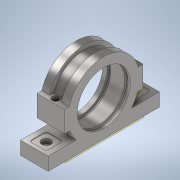
# Autodesk Inventor part: Корпус_Подшипника
Saved by Autodesk Inventor 2021 (Build 250183000, 183)
## iProperties
Created: 2023-04-25
Part Number: Корпус_Подшипника
Material: Сталь, углеродистая
Document SubType Name: Modeling
Designer: gdevc
Density: 7.85 g/cm^3
Appearance: С умеренной полировкой
Author: gdevc
Autodesk Inventor part; units mm, degrees
ref_plane "YZ Plane" through (0, 0, 0) normal (1, 0, 0) x (0, 1, 0)
ref_plane "XY Plane" through (0, 0, 0) normal (0, 0, 1) x (1, 0, 0)
sketch "Эскиз1" plane through (0, 0, 0) normal (0, 0, 1) x (1, 0, 0)
  line L0 (0, 0) -> (119.1589, 0)
  line L1 (0, 50) -> (52, 50)
  line L2 (52, 50) -> (52, 67.5)
  line L3 (0, 67.5) -> (0, 50)
  line L4 (0, 67.5) -> (15, 67.5)
  line L5 (15, 67.5) -> (15, 60)
  line L6 (15, 60) -> (37, 60)
  line L7 (37, 60) -> (37, 67.5)
  line L8 (37, 67.5) -> (52, 67.5)
  dimension "d0" = 100
  dimension "d1" = 52
  dimension "d2" = 135
  dimension "d3" = 10
  dimension "d4" = 15
  dimension "d5" = 15
  constraints: 18 end point, 5 perpendicular, 3 horizontal, 2 point on line
  measures "d0" diameter of L1 L0
  measures "d1" distance of L1.start L1.end
  measures "d2" diameter of L4 L0
  measures "d3" distance between parallel lines of L1 L6
  measures "d4" distance between parallel lines of L3 L5
  measures "d5" distance between parallel lines of L2 L7
revolve "Вращение1" add sketch "Эскиз1" angle 360 about axis through (0, 0, 0) along (1, 0, 0)
ref_plane "РабПлоскость1" through (0, -67.5, 0) normal (0, 1, 0) x (-1, 0, 0)
sketch "Эскиз3" plane through (0, -67.5, 0) normal (0, 1, 0) x (-1, 0, 0)
  line L0 (0, 0) -> (0, -105)
  line L1 (0, 67.5) -> (0, -67.5) projected
  line L2 (0, -105) -> (-52, -105)
  line L3 (-52, 67.5) -> (-52, -67.5) projected
  line L4 (-52, -105) -> (-52, 47.2217)
  line L5 (0, 105) -> (0, 0)
  line L6 (0, 105) -> (-52, 105)
  line L7 (-52, 105) -> (-52, 44.8764)
  dimension "d15" = 52
  dimension "d16" = 210
  dimension "d17" = 105
  constraints: 12 end point, 1 collinear, 1 horizontal, 1 parallel, 1 perpendicular, 1 point on line
  measures "d15" distance of L0.end L2.end
  measures "d16" distance between parallel lines of L6 L2
  measures "d17" distance from line of L0.start L2
extrude "Выдавливание1" add sketch "Эскиз3" along normal blind 25
sketch "Эскиз2" plane through (0, 0, 0) normal (0, 0, 1) x (1, 0, 0)
  line L0 (9, 50) -> (9, 54)
  line L1 (9, 54) -> (15, 54)
  line L2 (15, 54) -> (15, 50)
  line L3 (42, 50) -> (42, 54)
  line L4 (42, 54) -> (48, 54)
  line L5 (48, 54) -> (48, 50)
  line L6 (52, -67.5) -> (52, 67.5) projected
  line L7 (-10.4, 0) -> (62.4, 0) projected
  line L8 (15, 54) -> (15, 0)
  line L9 (15, -42.5) -> (15, 60) projected
  line L10 (9, 0) -> (9, 50)
  line L11 (48, 50) -> (48, 0)
  line L12 (48, 0) -> (42, 0)
  line L13 (42, 50) -> (42, 0)
  line L14 (52, 50) -> (0, 50) projected
  line L15 (9, 0) -> (15, 0)
  point P0 (0, 0)
  dimension "d7" = 54
  dimension "d8" = 6
  dimension "d9" = 9
  dimension "d10" = 4
  dimension "d11" = 54
  dimension "d12" = 6
  constraints: 24 end point, 5 perpendicular, 5 point on line, 2 vertical, 1 collinear
  measures "d7" distance from line of point (0, 0) L1
  measures "d8" distance between parallel lines of L2 L0
  measures "d9" distance from line of point (0, 0) L0
  measures "d10" distance between parallel lines of L6 L5
  measures "d11" distance from line of point (0, 0) L4
  measures "d12" distance between parallel lines of L5 L3
revolve "Вращение2" cut sketch "Эскиз2" angle 360 about axis through (-10, 0, 0) along (1, 0, 0) contours L14 L8 L7 L10 | L0 L1 L2 L14 | L14 L11 L7 L13 | L3 L4 L5 L14
sketch "Эскиз4" plane through (0, -67.5, -105) normal (-1, 0, 0) x (0, 0, 1)
  arc A0 (131.3391, 25) -> (78.6609, 25) centre (105, 67.5) ccw projected
  arc A1 (157.4404, 25) -> (52.5596, 25) centre (105, 67.5) ccw projected
  circle A2 centre (105, 67.5) radius 50
  point P0 (78.6609, 25)
  constraints: 1 centre point, 1 coincident
extrude "Выдавливание2" cut sketch "Эскиз4" against normal through all
ref_plane "РабПлоскость2" through (0, -42.5, 0) normal (0, 1, 0) x (-1, 0, 0)
sketch "Эскиз5" plane through (0, -42.5, 0) normal (0, 1, 0) x (-1, 0, 0)
  line L0 (-37, -98.5) -> (-15, -98.5)
  line L1 (-10, -93.5) -> (-10, -71.5)
  line L2 (-15, -66.5) -> (-37, -66.5)
  line L3 (-42, -71.5) -> (-42, -93.5)
  line L4 (-42, -82.5) -> (-10, -82.5) construction
  arc A0 (-42, -93.5) -> (-37, -98.5) centre (-37, -93.5) ccw
  arc A1 (-15, -98.5) -> (-10, -93.5) centre (-15, -93.5) ccw
  arc A2 (-10, -71.5) -> (-15, -66.5) centre (-15, -71.5) ccw
  arc A3 (-37, -66.5) -> (-42, -71.5) centre (-37, -71.5) ccw
  circle A4 centre (-26, -82.5) radius 8.5
  line L5 (-80.9956, 0) -> (7.5507, 0) construction
  line L6 (-37, 98.5) -> (-15, 98.5)
  line L7 (-10, 93.5) -> (-10, 71.5)
  line L8 (-15, 66.5) -> (-37, 66.5)
  line L9 (-42, 71.5) -> (-42, 93.5)
  line L10 (-42, 82.5) -> (-10, 82.5) construction
  arc A5 (-37, 98.5) -> (-42, 93.5) centre (-37, 93.5) ccw
  arc A6 (-10, 93.5) -> (-15, 98.5) centre (-15, 93.5) ccw
  arc A7 (-15, 66.5) -> (-10, 71.5) centre (-15, 71.5) ccw
  arc A8 (-42, 71.5) -> (-37, 66.5) centre (-37, 71.5) ccw
  circle A9 centre (-26, 82.5) radius 8.5
  point P0 (0, 0)
  dimension "d23" = 165
  dimension "d24" = 32
  dimension "d25" = 32
  dimension "d26" = 10
  dimension "d27" = 5
  dimension "d28" = 17
  constraints: 22 end point, 16 point on circle, 15 symmetric about line, 10 centre point, 8 tangent, 3 equal radius, 3 midpoint, 2 horizontal, 2 parallel, 1 perpendicular, 5 other
  measures "d23" diameter of point (0, 0) L4
  measures "d24" distance between parallel lines of L2 L0
  measures "d25" distance between parallel lines of L3 L1
  measures "d26" distance from line of point (0, 0) L1
  measures "d27" radius of A0
  measures "d28" diameter of A4
extrude "Выдавливание3" cut sketch "Эскиз5" against normal blind 1
extrude "Выдавливание4" cut sketch "Эскиз5" against normal through all contours A4 | A9
ref_plane "РабПлоскость3" through (26, -67.5, -105) normal (-1, 0, 0) x (0, 0, 1)
sketch "Эскиз6" plane through (26, -67.5, -105) normal (-1, 0, 0) x (0, 0, 1)
  line L0 (210, 0) -> (0, 0) projected
  line L1 (7.5, 15) -> (37.5, 15)
  line L2 (37.5, 15) -> (37.5, 0)
  line L3 (37.5, 0) -> (7.5, 0)
  line L4 (7.5, 0) -> (7.5, 15)
  line L5 (31, 24) -> (14, 24) projected
  line L6 (31, 0) -> (14, 0) projected
  line L7 (31, 0) -> (14, 0) projected
  line L8 (22.5, 0) -> (22.5, 18.5711) construction
  line L9 (105, 67.5) -> (105, 0) construction
  line L10 (0, 0) -> (210, 0)
  line L11 (202.5, 15) -> (172.5, 15)
  line L12 (172.5, 15) -> (172.5, 0)
  line L13 (202.5, 0) -> (202.5, 15)
  point P0 (202.5, 0)
  point P1 (7.5, 0)
  dimension "d34" = 30
  dimension "d35" = 30
  dimension "d36" = 15
  constraints: 20 end point, 6 symmetric about line, 2 midpoint, 2 parallel, 2 point on line, 1 horizontal, 1 perpendicular, 1 vertical
  measures "d34" distance between parallel lines of L2 L4
  measures "d35" diameter of L4 L8
  measures "d36" distance between parallel lines of L0 L1
extrude "Выдавливание5" cut sketch "Эскиз6" along normal mid plane 42
ref_plane "РабПлоскость4" through (0, 18.5, 0) normal (0, 1, 0) x (-1, 0, 0)
sketch "Эскиз9" plane through (0, -67.5, -105) normal (-1, 0, 0) x (0, 0, 1)
  line L0 (-42, 86) -> (252, 86) projected
  arc A0 (157.4404, 25) -> (52.5596, 25) centre (105, 67.5) ccw projected
  arc A1 (147.3527, 25) -> (62.6473, 25) centre (105, 67.5) ccw projected
  line L1 (40.0847, 86) -> (31, 86)
  line L2 (31, 86) -> (31, 46)
  line L3 (31, 46) -> (41.0156, 46)
  line L4 (7.5, 15) -> (37.5, 15) projected
  line L5 (31, 24) -> (14, 24) projected
  dimension "d46" = 40
  constraints: 6 end point, 3 point on line, 2 point on circle, 1 perpendicular, 1 vertical
  measures "d46" distance of L1.end L2.end
extrude "Выдавливание7" add sketch "Эскиз9" against normal blind 15 contours L0 A0 L3 L2
sketch "Эскиз10" plane through (26, -67.5, -105) normal (-1, 0, 0) x (0, 0, 1)
  line L0 (31, 46) -> (31, 86) projected
  line L1 (157.4404, 25) -> (147.3527, 25) projected
  arc A0 (147.3527, 25) -> (62.6473, 25) centre (105, 67.5) ccw projected
  line L2 (62.6473, 25) -> (52.5596, 25) projected
  arc A1 (41.0156, 46) -> (52.5596, 25) centre (105, 67.5) ccw projected
  line L3 (41.0156, 46) -> (31, 46) projected
  line L4 (31, 46) -> (31, 86) projected
  line L5 (31, 86) -> (40.0847, 86) projected
  arc A2 (157.4404, 25) -> (40.0847, 86) centre (105, 67.5) ccw projected
  arc A3 (147.3527, 25) -> (62.6473, 25) centre (105, 67.5) ccw projected
  line L6 (31, 86) -> (47.9233, 86)
  line L7 (31, 46) -> (41.0156, 46) projected
  line L8 (31, 46) -> (48.9844, 46)
  line L9 (105, 67.5) -> (105, 135) construction
  arc A4 (157.4404, 25) -> (40.0847, 86) centre (105, 67.5) ccw projected
  line L10 (179, 46) -> (179, 86)
  line L11 (168.9844, 46) -> (179, 46)
  line L12 (179, 46) -> (179, 86)
  line L13 (179, 86) -> (169.9153, 86)
  line L14 (179, 86) -> (162.0767, 86)
  line L15 (179, 46) -> (168.9844, 46)
  line L16 (179, 46) -> (161.0156, 46)
  point P0 (41.0156, 46)
  constraints: 20 end point, 8 symmetric about line, 3 point on circle, 1 collinear, 1 horizontal, 1 vertical
extrude "Выдавливание8" add sketch "Эскиз10" along normal mid plane 52 contours L0 L5 L6 A0 L8 L3 | L13 L10 L11 A2
ref_plane "РабПлоскость5" through (26, -67.5, 105) normal (1, 0, 0) x (0, 0, -1)
sketch "Эскиз11" plane through (26, -67.5, 105) normal (1, 0, 0) x (0, 0, -1)
  arc A0 (162.0767, 86) -> (62.6473, 25) centre (105, 67.5) ccw projected
  line L0 (31, 86) -> (40.0847, 86) projected
  line L1 (47.9233, 86) -> (31, 86)
  line L2 (31, 46) -> (31, 86) projected
  line L3 (31, 86) -> (31, 46)
  line L4 (31, 46) -> (48.9844, 46)
  arc A1 (47.9233, 86) -> (48.9844, 46) centre (105, 67.5) ccw
  constraints: 6 end point, 4 point on circle, 2 collinear, 1 centre point, 1 coincident, 1 perpendicular
extrude "Выдавливание9" add sketch "Эскиз11" along normal mid plane 52
sketch "Эскиз12" plane through (15, 18.5, -57.0767) normal (0, 1, 0) x (1, 0, 0)
  line L0 (0, 4.7941) -> (0, -1.0611) projected
  line L1 (22, -1.0611) -> (22, 6.9077) projected
  line L2 (-15, 16.9233) -> (37, 16.9233) projected
  line L3 (37, 6.9077) -> (37, 16.9233) projected
  line L4 (22, 6.9077) -> (37, 6.9077) projected
  line L5 (22, -1.0611) -> (22, 6.9077) projected
  line L6 (0, -1.0611) -> (22, -1.0611) projected
  line L7 (0, 6.9077) -> (0, -1.0611) projected
  line L8 (-15, 6.9077) -> (0, 6.9077) projected
  line L9 (0, -121.0611) -> (-15, -121.0611) projected
  line L10 (0, -113.0923) -> (0, -121.0611) projected
  line L11 (22, -113.0923) -> (0, -113.0923) projected
  line L12 (22, -121.0611) -> (22, -113.0923) projected
  line L13 (37, -121.0611) -> (22, -121.0611) projected
  circle A0 centre (11, 7.9389) radius 6.5
  line L14 (37, -107.0767) -> (37, -7.0767) projected
  line L15 (37, -57.0767) -> (-15, -57.0767) construction
  circle A1 centre (11, -122.0923) radius 6.5
  line L16 (37, -131.0767) -> (-15, -131.0767) projected
  line L17 (-15, -121.0611) -> (-15, -131.0767) projected
  line L18 (37, -131.0767) -> (37, -121.0611) projected
  line L19 (-15, 16.9233) -> (-15, 6.9077) projected
  dimension "d61" = 13
  dimension "d62" = 11
  dimension "d63" = 9
  constraints: 2 centre point, 2 end point, 1 horizontal, 1 midpoint, 1 symmetric about line, 1 other
  measures "d61" diameter of A0
  measures "d62" distance from line of L1 A0.centre
  measures "d63" distance from line of L6 A0.centre
ref_plane "РабПлоскость6" through (0, -21.5, -64.9153) normal (0, 1, 0) x (1, 0, 0)
sketch "Эскиз13" plane through (0, -21.5, -64.9153) normal (0, 1, 0) x (1, 0, 0)
  circle A0 centre (26, 0.1003) radius 6.5 projected
  circle A1 centre (26, -129.931) radius 6.5 projected
  circle A2 centre (26, 0.1003) radius 6
  circle A3 centre (26, -129.931) radius 6
  point P0 (0, -64.9153)
  dimension "d65" = 12
  dimension "d66" = 12
  constraints: 2 centre point, 2 coincident
  measures "d65" diameter of A2
  measures "d66" diameter of A3
extrude "Выдавливание10" cut sketch "Эскиз13" along normal blind 10 contours A2 | A3
thread "Резьба1" size "M12x1.75" class "6H" standard "ANSI Metric M Profile" length 18
thread "Резьба2" size "M12x1.75" class "6H" standard "ANSI Metric M Profile" length 18
extrude "Выдавливание11" cut sketch "Эскиз12" against normal blind 30 contours A0 | A1
equation "\"d17\" = 0.5 * d16"
equation "\"d35\" = d34"
